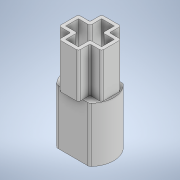
# Autodesk Inventor part: motor-lego-adapter-3-4
Saved by Autodesk Inventor 2020 (Build 240168000, 168)
## iProperties
Created: 2023-04-25
Part Number: motor-lego-adapter-3-4
Material: Generic
Document SubType Name: Modeling
Designer: 22hamfri
Density: 1 g/cm^3
Appearance: Default
Author: 22hamfri
Autodesk Inventor part; units mm, degrees
ref_plane "YZ Plane" through (0, 0, 0) normal (1, 0, 0) x (0, 1, 0)
ref_plane "XZ Plane" through (0, 0, 0) normal (0, 1, 0) x (-1, 0, 0)
ref_plane "XY Plane" through (0, 0, 0) normal (0, 0, 1) x (1, 0, 0)
sketch "Sketch1" plane through (0, 0, 0) normal (0, 1, 0) x (-1, 0, 0)
  line L0 (-2.85, 1.9) -> (2.85, 1.9)
  line L1 (2.85, 1.9) -> (2.85, -1.9)
  line L2 (2.85, -1.9) -> (-2.85, -1.9)
  line L3 (-2.85, -1.9) -> (-2.85, 1.9)
  line L4 (-2.85, 1.9) -> (2.85, -1.9) construction
  line L5 (2.85, 1.9) -> (-2.85, -1.9) construction
  line L6 (3.45, -2.5) -> (3.45, 2.5)
  line L7 (3.45, 2.5) -> (-3.45, 2.5)
  line L8 (-3.45, 2.5) -> (-3.45, -2.5)
  line L9 (-3.45, -2.5) -> (3.45, -2.5)
  circle A0 centre (0, 0) radius 2.85
  circle A1 centre (0, 0) radius 3.45
  point P0 (-2.1243, 1.9)
  point P1 (2.1243, 1.9)
  point P2 (2.1243, -1.9)
  point P3 (-2.1243, -1.9)
  point P4 (-2.3775, 2.5)
  point P5 (-2.3775, -2.5)
  point P6 (2.3775, -2.5)
  point P7 (2.3775, 2.5)
  dimension "d0" = 3.8
  dimension "d1" = 0.6
  dimension "d2" = 5.7
  constraints: 20 end point, 4 parallel, 2 centre point, 2 coincident, 2 midpoint, 2 perpendicular, 2 tangent, 1 horizontal, 3 other
  measures "d0" distance between parallel lines of L2 L0
  measures "d1" distance between parallel lines of L9 L2
  measures "d2" distance of L1.end L2.end
extrude "Extrusion1" add sketch "Sketch1" along normal blind 7.5 contours L3 L2 A0 L9 A1 L7 L0 | L0 A0 L3 | A0 L7 L0 | A0 L2 L3 | A0 L7 A1 L9 L2 L1 L0 | L0 L1 A0 | L2 A0 L9 | L1 L2 A0
sketch "Sketch2" plane through (0, 7.5, 0) normal (0, 1, 0) x (1, 0, 0)
  arc A0 (2.3775, -2.5) -> (2.3775, 2.5) centre (0, 0) ccw projected
  line L0 (2.3775, 2.5) -> (-2.3775, 2.5) projected
  arc A1 (-2.3775, 2.5) -> (-2.3775, -2.5) centre (0, 0) ccw projected
  line L1 (-2.3775, -2.5) -> (2.3775, -2.5) projected
  arc A2 (2.1243, -1.9) -> (2.1243, 1.9) centre (0, 0) ccw projected
  line L2 (2.1243, -1.9) -> (-2.1243, -1.9) projected
  arc A3 (-2.1243, 1.9) -> (-2.1243, -1.9) centre (0, 0) ccw projected
  line L3 (-2.1243, 1.9) -> (2.1243, 1.9) projected
extrude "Extrusion2" add sketch "Sketch2" along normal blind 0.5 contours L1 A1 L0 A0 | L2 A3 L3 A2
sketch "Sketch3" plane through (0, 8, 0) normal (0, 1, 0) x (1, 0, 0)
  line L0 (-0.925, -2.625) -> (-0.925, 2.625)
  line L1 (-0.925, 2.625) -> (0.925, 2.625)
  line L2 (0.925, 2.625) -> (0.925, -2.625)
  line L3 (0.925, -2.625) -> (-0.925, -2.625)
  line L4 (-0.925, -2.625) -> (0.925, 2.625) construction
  line L5 (-0.925, 2.625) -> (0.925, -2.625) construction
  line L6 (-2.625, -0.925) -> (2.625, -0.925)
  line L7 (2.625, -0.925) -> (2.625, 0.925)
  line L8 (2.625, 0.925) -> (-2.625, 0.925)
  line L9 (-2.625, 0.925) -> (-2.625, -0.925)
  line L10 (-2.625, -0.925) -> (2.625, 0.925) construction
  line L11 (2.625, -0.925) -> (-2.625, 0.925) construction
  line L12 (-3.125, 1.425) -> (3.125, 1.425)
  line L13 (3.125, 1.425) -> (3.125, -1.425)
  line L14 (3.125, -1.425) -> (-3.125, -1.425)
  line L15 (-3.125, -1.425) -> (-3.125, 1.425)
  line L16 (1.425, -3.125) -> (1.425, 3.125)
  line L17 (1.425, 3.125) -> (-1.425, 3.125)
  line L18 (-1.425, 3.125) -> (-1.425, -3.125)
  line L19 (-1.425, -3.125) -> (1.425, -3.125)
  point P0 (0, 0)
  point P1 (-1.425, -1.425)
  point P2 (1.425, -1.425)
  point P3 (1.425, 1.425)
  point P4 (-1.425, 1.425)
  dimension "d7" = 5.25
  dimension "d8" = 5.25
  dimension "d9" = 1.85
  dimension "d10" = 1.85
  dimension "d11" = 0.5
  dimension "d12" = 0.5
  constraints: 40 end point, 8 parallel, 4 midpoint, 4 perpendicular, 1 horizontal, 1 vertical, 6 other
  measures "d7" distance between parallel lines of L7 L9
  measures "d8" distance between parallel lines of L3 L1
  measures "d9" distance of L2.end L0.start
  measures "d10" distance of L6.end L7.end
  measures "d11" distance between parallel lines of L7 L13
  measures "d12" distance between parallel lines of L16 L2
extrude "Extrusion3" add sketch "Sketch3" along normal blind 0.5
sketch "Sketch4" plane through (0, 8.5, 0) normal (0, 1, 0) x (1, 0, 0)
  line L0 (-3.125, 1.425) -> (-3.125, -1.425) projected
  line L1 (-3.125, -1.425) -> (-1.425, -1.425) projected
  line L2 (-1.425, -1.425) -> (-1.425, -3.125) projected
  line L3 (-1.425, -3.125) -> (1.425, -3.125) projected
  line L4 (1.425, -3.125) -> (1.425, -1.425) projected
  line L5 (1.425, -1.425) -> (3.125, -1.425) projected
  line L6 (3.125, -1.425) -> (3.125, 1.425) projected
  line L7 (3.125, 1.425) -> (1.425, 1.425) projected
  line L8 (1.425, 1.425) -> (1.425, 3.125) projected
  line L9 (1.425, 3.125) -> (-1.425, 3.125) projected
  line L10 (-1.425, 3.125) -> (-1.425, 1.425) projected
  line L11 (-1.425, 1.425) -> (-3.125, 1.425) projected
  line L12 (-2.625, -0.925) -> (-2.625, 0.925)
  line L13 (-2.625, 0.925) -> (-0.925, 0.925)
  line L14 (-0.925, 0.925) -> (-0.925, 2.625)
  line L15 (-0.925, 2.625) -> (0.925, 2.625)
  line L16 (0.925, 2.625) -> (0.925, 0.925)
  line L17 (0.925, 0.925) -> (2.625, 0.925)
  line L18 (2.625, 0.925) -> (2.625, -0.925)
  line L19 (2.625, -0.925) -> (0.925, -0.925)
  line L20 (0.925, -0.925) -> (0.925, -2.625)
  line L21 (0.925, -2.625) -> (-0.925, -2.625)
  line L22 (-0.925, -2.625) -> (-0.925, -0.925)
  line L23 (-0.925, -0.925) -> (-2.625, -0.925)
  point P0 (0, 0)
  dimension "d15" = 0.5
  constraints: 24 end point, 11 other
  measures "d15" distance between parallel lines of L11 L13
extrude "Extrusion4" add sketch "Sketch4" along normal blind 6
fillet "Fillet1" radius 0.3 8 edges at (1.425, 11.25, 3.125) (3.125, 11.25, 1.425) (3.125, 11.25, -1.425) (1.425, 11.25, -3.125) (-1.425, 11.25, -3.125) (-3.125, 11.25, -1.425) (-1.425, 11.25, 3.125) (-3.125, 11.25, 1.425)
fillet "Fillet2" radius 0.3 4 edges at (-0.925, 11.5, 0.925) (0.925, 11.5, 0.925) (0.925, 11.5, -0.925) (-0.925, 11.5, -0.925)
fillet "Fillet3" radius 0.5 4 edges at (2.3775, 4, -2.5) (-2.3775, 4, -2.5) (-2.3775, 4, 2.5) (2.3775, 4, 2.5)
sketch "Sketch5" plane through (0, 8.5, 0) normal (0, 1, 0) x (1, 0, 0)
  line L0 (2.625, 0.925) -> (1.225, 0.925) projected
  arc A0 (0.925, 1.225) -> (1.225, 0.925) centre (1.225, 1.225) ccw projected
  line L1 (0.925, 1.225) -> (0.925, 2.625) projected
  line L2 (0.925, 2.625) -> (-0.925, 2.625) projected
  line L3 (-0.925, 2.625) -> (-0.925, 1.225) projected
  arc A1 (-1.225, 0.925) -> (-0.925, 1.225) centre (-1.225, 1.225) ccw projected
  line L4 (-1.225, 0.925) -> (-2.625, 0.925) projected
  line L5 (-2.625, 0.925) -> (-2.625, -0.925) projected
  line L6 (-2.625, -0.925) -> (-1.225, -0.925) projected
  arc A2 (-0.925, -1.225) -> (-1.225, -0.925) centre (-1.225, -1.225) ccw projected
  line L7 (-0.925, -1.225) -> (-0.925, -2.625) projected
  line L8 (-0.925, -2.625) -> (0.925, -2.625) projected
  line L9 (0.925, -2.625) -> (0.925, -1.225) projected
  arc A3 (1.225, -0.925) -> (0.925, -1.225) centre (1.225, -1.225) ccw projected
  line L10 (1.225, -0.925) -> (2.625, -0.925) projected
  line L11 (2.625, -0.925) -> (2.625, 0.925) projected
  line L12 (-2.1243, 1.9) -> (2.1243, 1.9) projected
  arc A4 (2.1243, -1.9) -> (2.1243, 1.9) centre (0, 0) ccw projected
  line L13 (2.1243, -1.9) -> (-2.1243, -1.9) projected
  arc A5 (-2.1243, 1.9) -> (-2.1243, -1.9) centre (0, 0) ccw projected
  point P0 (2.5898, -0.925)
  point P1 (2.625, -0.8197)
  point P2 (2.625, 0.8197)
  point P3 (2.5898, 0.925)
  point P4 (0.925, 1.9)
  point P5 (-0.925, 1.9)
  point P6 (-2.5898, 0.925)
  point P7 (-2.625, 0.8197)
  point P8 (-2.625, -0.8197)
  point P9 (-2.5898, -0.925)
  point P10 (-0.925, -1.9)
  point P11 (0.925, -1.9)
extrude "Extrusion5" cut sketch "Sketch5" against normal up to surface (1 mm away) contours L11 L10 A3 L9 L13 L7 A2 L6 L5 L4 A1 L3 L12 L1 A0 L0
fillet "Fillet4" radius 0.2 4 edges at (-1.425, 11.25, 1.425) (1.425, 11.25, 1.425) (1.425, 11.25, -1.425) (-1.425, 11.25, -1.425)
equation "\"d8\" = d7"
equation "\"d10\" = d9"
equation "\"d12\" = d11"
equation "\"d15\" = d11"
body "Solid1"
